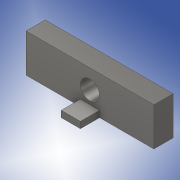
# Autodesk Inventor part: C005
Saved by Autodesk Inventor 2017 (Build 210142000, 142)
## iProperties
Created: 2017-06-13
Part Number: C005
Material: Steel, Carbon
Document SubType Name: Modeling
Designer: zallen
Density: 7.85 g/cm^3
Appearance: Semi-Polished
Author: zallen
Autodesk Inventor part; units mm, degrees
ref_plane "YZ Plane" through (0, 0, 0) normal (1, 0, 0) x (0, 1, 0)
ref_plane "XZ Plane" through (0, 0, 0) normal (0, 1, 0) x (-1, 0, 0)
ref_plane "XY Plane" through (0, 0, 0) normal (0, 0, 1) x (1, 0, 0)
sketch "Sketch1" plane through (0, 0, 0) normal (0, 0, 1) x (1, 0, 0)
  line L0 (0, 0) -> (100, 0)
  circle A0 centre (50, 15) radius 7.5
  line L1 (0, 0) -> (0, 30)
  line L2 (0, 30) -> (100, 30)
  line L3 (100, 30) -> (100, 0)
  point P0 (50, 0)
  dimension "d0" = 100
  dimension "d2" = 15
  dimension "d3" = 15
  dimension "d4" = 30
  constraints: 8 end point, 2 perpendicular, 1 centre point, 1 horizontal, 1 midpoint, 1 vertical, 1 vertical alignment
  measures "d0" distance of L0.start L0.end
  measures "d2" diameter of A0
  measures "d3" distance of point (50, 0) A0.centre
  measures "d4" distance of L0.start L1.end
extrude "Extrusion1" add sketch "Sketch1" along normal blind 15
sketch "Sketch2" plane through (0, 0, 15) normal (0, 0, 1) x (1, 0, 0)
  line L0 (0, 0) -> (100, 0) projected
  line L1 (42.5, 0) -> (57.5, 0)
  line L2 (57.5, 0) -> (57.5, 5)
  line L3 (57.5, 5) -> (42.5, 5)
  line L4 (42.5, 5) -> (42.5, 0)
  point P0 (50, 0)
  dimension "d7" = 15
  dimension "d8" = 5
  constraints: 8 end point, 2 midpoint, 2 parallel, 1 horizontal, 1 perpendicular, 1 point on line
  measures "d7" distance of L3.end L2.end
  measures "d8" distance of L1.end L2.end
extrude "Extrusion2" add sketch "Sketch2" along normal blind 15
body "Solid1"
